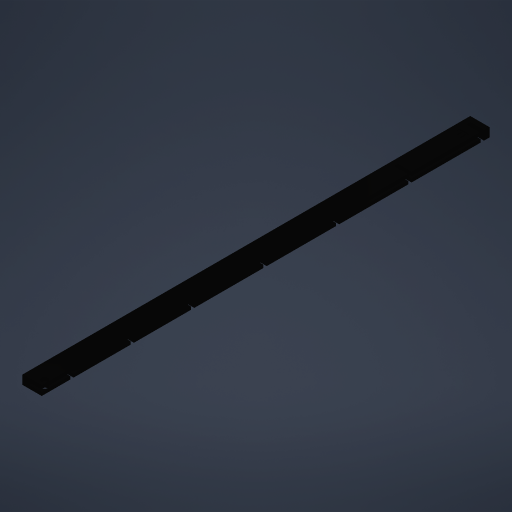
# Autodesk Inventor part: Jig_1
Saved by Autodesk Inventor 2023 (Build 270158000, 158)
## iProperties
Created: 2023-05-07
Part Number: Jig_1
Material: Generic
Document SubType Name: Modeling
Designer: szykr
Density: 1 g/cm^3
Appearance: Anodized - Black
Author: szykr
Autodesk Inventor part; units mm, degrees
ref_plane "YZ Plane" through (0, 0, 0) normal (1, 0, 0) x (0, 1, 0)
ref_plane "XZ Plane" through (0, 0, 0) normal (0, 1, 0) x (-1, 0, 0)
ref_plane "XY Plane" through (0, 0, 0) normal (0, 0, 1) x (1, 0, 0)
sketch "Sketch1" plane through (0, 0, 0) normal (0, 1, 0) x (-1, 0, 0)
  line L0 (34.2517, -400) -> (39.9859, -400) projected
  line L1 (39.9859, -398.5) -> (34.2517, -398.5) projected
  line L2 (40, -362.5) -> (40, -400) projected
  line L3 (-17.5197, -362.5) -> (39.9985, -362.5) projected
  line L4 (-17.5197, -361) -> (39.9985, -361) projected
  line L5 (-30.0427, -325) -> (39.9996, -325) projected
  line L6 (-30.0427, -323.5) -> (39.9996, -323.5) projected
  line L7 (-37.5246, -287.5) -> (39.9992, -287.5) projected
  line L8 (-37.5246, -286) -> (39.9992, -286) projected
  line L9 (-40, -250) -> (40, -250) projected
  line L10 (40, -248.5) -> (-40, -248.5) projected
  line L11 (-40, -218.75) -> (40, -218.75) projected
  line L12 (40, -217.25) -> (-40, -217.25) projected
  line L13 (-40, -187.5) -> (40, -187.5) projected
  line L14 (40, -186) -> (-40, -186) projected
  line L15 (-40, -156.25) -> (40, -156.25) projected
  line L16 (40, -154.75) -> (-40, -154.75) projected
  line L17 (-40, -125) -> (40, -125) projected
  line L18 (40, -123.5) -> (-40, -123.5) projected
  line L19 (-40, -93.75) -> (40, -93.75) projected
  line L20 (40, -92.25) -> (-40, -92.25) projected
  line L21 (-40, -62.5) -> (40, -62.5) projected
  line L22 (40, -61) -> (-40, -61) projected
  line L23 (-20.0599, -31.25) -> (40, -31.25) projected
  line L24 (40, -29.75) -> (-20.0599, -29.75) projected
  line L25 (-22.1824, 0) -> (40, 0) projected
  line L26 (40, 1.5) -> (-22.1824, 1.5) projected
  line L27 (-25.7924, 37.5) -> (37.5967, 37.5) projected
  line L28 (-25.7924, 39) -> (37.5967, 39) projected
  line L29 (-27.8365, 75) -> (30.1757, 75) projected
  line L30 (-27.8365, 76.5) -> (30.1757, 76.5) projected
  spline S0 degree 3 poles (-27.5913, 112.5) (-26.0233, 112.5) (-24.3482, 112.5) (-19.9699, 112.5) (-17.1747, 112.5) (-12.6594, 112.5) (-11.0052, 112.5) (-5.6992, 112.5) (-2.1464, 112.5) (4.6917, 112.5) (7.898, 112.5) (12.94, 112.5) (14.8552, 112.5) (17.0133, 112.5) (17.7292, 112.5) (17.4374, 112.5) (16.5312, 112.5) (13.3266, 112.5) (10.8916, 112.5) (5.1483, 112.5) (1.9055, 112.5) (-4.6814, 112.5) (-7.9404, 112.5) (-11.2251, 112.5) knots -12.727759 -12.727759 -12.727759 -12.727759 -11.944404 -11.944404 -10.775364 -10.775364 -10.102311 -10.102311 -8.634698 -8.634698 -7.023718 -7.023718 -5.528611 -5.528611 -4.394104 -4.394104 -3.316195 -3.316195 -2.113862 -2.113862 -0.985401 -0.985401 0 0 0 0 projected
  spline S1 degree 3 poles (-11.2251, 114) (-7.9404, 114) (-4.6814, 114) (1.9055, 114) (5.1483, 114) (10.8916, 114) (13.3266, 114) (16.5312, 114) (17.4374, 114) (17.7292, 114) (17.0133, 114) (14.8552, 114) (12.94, 114) (7.898, 114) (4.6917, 114) (-2.1464, 114) (-5.6992, 114) (-11.0052, 114) (-12.6594, 114) (-17.1747, 114) (-19.9699, 114) (-24.3482, 114) (-26.0233, 114) (-27.5913, 114) knots 0 0 0 0 0.985401 0.985401 2.113862 2.113862 3.316195 3.316195 4.394104 4.394104 5.528611 5.528611 7.023718 7.023718 8.634698 8.634698 10.102311 10.102311 10.775364 10.775364 11.944404 11.944404 12.727759 12.727759 12.727759 12.727759 projected
  line L31 (-40, 150) -> (0, 150) projected
  line L32 (0, 151.5) -> (-40, 151.5) projected
  line L33 (40, -325) -> (40, -361) projected
  line L34 (40, -287.5) -> (40, -323.5) projected
  line L35 (40, -250) -> (40, -286) projected
  line L36 (40, -218.75) -> (40, -248.5) projected
  line L37 (40, -187.5) -> (40, -217.25) projected
  line L38 (40, -171.125) -> (40, -186) projected
  line L39 (42.9859, -400) -> (42.9859, -171.125)
  line L40 (42.9859, -400) -> (40, -400)
  line L41 (40, -171.125) -> (42.9859, -171.125)
  line L42 (32.9859, -400) -> (32.9859, -171.125)
  line L43 (32.9859, -400) -> (40, -400)
  line L44 (32.9859, -171.125) -> (40, -171.125)
  line L45 (40, -325) -> (40, -323.5)
  line L46 (40, -287.5) -> (40, -286)
  line L47 (40, -250) -> (40, -248.5)
  line L48 (40, -218.75) -> (40, -217.25)
  line L49 (40, -187.5) -> (40, -186)
  line L50 (42.9859, -400) -> (42.9859, -403)
  line L51 (42.9859, -403) -> (32.9859, -403)
  line L52 (32.9859, -403) -> (32.9859, -400)
  line L53 (34.2517, -398.5) -> (32.9859, -398.5)
  line L54 (40, -362.5) -> (39.9985, -362.5)
  line L55 (40, -362.5) -> (40, -361)
  line L56 (39.9985, -361) -> (40, -361)
  line L57 (39.9992, -287.5) -> (40, -287.5)
  line L58 (39.9992, -286) -> (40, -286)
  line L59 (39.9996, -323.5) -> (40, -323.5)
  line L60 (39.9996, -325) -> (40, -325)
  point P0 (0, 0)
  point P1 (41.493, -400)
  dimension "d2" = 3
  dimension "d5" = 10
  dimension "d6" = 3
  constraints: 44 end point, 7 horizontal, 5 collinear, 5 perpendicular, 4 vertical, 1 horizontal alignment, 1 midpoint, 1 parallel, 1 point on line
  measures "d2" distance from line of L39 L0.end
  measures "d5" distance between parallel lines of L39 L42
  measures "d6" distance of L39.start L50.end
extrude "Extrusion1" add sketch "Sketch1" along normal mid plane 1.6 contours L0 L43 L40 L50 L51 L52 | L2 L55 L33 L45 L34 L46 L35 L47 L36 L48 L37 L49 L38 L41 L39 L40
sketch "Sketch2" plane through (0, 0.8, 0) normal (0, 1, 0) x (1, 0, 0)
  circle A0 centre (-35, 174.625) radius 1.5 projected
  line L0 (-40, 171.125) -> (-30, 171.125) projected
  line L1 (-30, 400) -> (-30, 171.125) projected
  line L2 (-40, 400) -> (-30, 400) projected
  line L3 (-40, 362.5) -> (-40, 400) projected
  line L4 (-35, 362.5) -> (-40, 362.5) projected
  line L5 (-35, 361) -> (-35, 362.5) projected
  line L6 (-40, 361) -> (-35, 361) projected
  line L7 (-40, 325) -> (-40, 361) projected
  line L8 (-34.9779, 325) -> (-40, 325) projected
  line L9 (-34.9779, 323.5) -> (-34.9779, 325) projected
  line L10 (-40, 323.5) -> (-34.9779, 323.5) projected
  line L11 (-40, 287.5) -> (-40, 323.5) projected
  line L12 (-35, 287.5) -> (-40, 287.5) projected
  line L13 (-35, 286) -> (-35, 287.5) projected
  line L14 (-40, 286) -> (-35, 286) projected
  line L15 (-40, 250) -> (-40, 286) projected
  line L16 (-35, 250) -> (-40, 250) projected
  line L17 (-35, 248.5) -> (-35, 250) projected
  line L18 (-40, 248.5) -> (-35, 248.5) projected
  line L19 (-40, 218.75) -> (-40, 248.5) projected
  line L20 (-35, 218.75) -> (-40, 218.75) projected
  line L21 (-35, 217.25) -> (-35, 218.75) projected
  line L22 (-40, 217.25) -> (-35, 217.25) projected
  line L23 (-40, 187.5) -> (-40, 217.25) projected
  line L24 (-35, 187.5) -> (-40, 187.5) projected
  line L25 (-35, 186) -> (-35, 187.5) projected
  line L26 (-40, 186) -> (-35, 186) projected
  line L27 (-40, 171.125) -> (-40, 186) projected
  line L28 (-32.9859, 403) -> (-42.9859, 403) projected
  line L29 (-42.9859, 403) -> (-42.9859, 171.125) projected
  line L30 (-32.9859, 400) -> (-32.9859, 403) projected
  line L31 (-42.9859, 171.125) -> (-40, 171.125) projected
  line L32 (-40, 400) -> (-32.9859, 400) projected
  line L33 (-32.9859, 400) -> (-32.9859, 171.125)
  line L34 (-35, 362.5) -> (-32.9859, 362.5)
  line L35 (-35, 361) -> (-32.9859, 361)
  line L36 (-34.9779, 325) -> (-32.9859, 325)
  line L37 (-34.9779, 323.5) -> (-32.9859, 323.5)
  line L38 (-35, 287.5) -> (-32.9859, 287.5)
  line L39 (-35, 286) -> (-32.9859, 286)
  line L40 (-35, 250) -> (-32.9859, 250)
  line L41 (-35, 248.5) -> (-32.9859, 248.5)
  line L42 (-35, 218.75) -> (-32.9859, 218.75)
  line L43 (-35, 217.25) -> (-32.9859, 217.25)
  line L44 (-35, 187.5) -> (-32.9859, 187.5)
  line L45 (-35, 186) -> (-32.9859, 186)
  line L46 (-40, 362.5) -> (-40, 361)
  line L47 (-40, 171.125) -> (-40, 400) projected
  line L48 (-40, 325) -> (-40, 323.5)
  line L49 (-40, 287.5) -> (-40, 286)
  line L50 (-40, 250) -> (-40, 248.5)
  line L51 (-40, 218.75) -> (-40, 217.25)
  line L52 (-40, 187.5) -> (-40, 186)
  line L53 (-39.9859, 398.5) -> (-34.2517, 398.5) projected
  line L54 (-34.2517, 398.5) -> (-32.9859, 398.5)
  line L55 (-39.9859, 398.5) -> (-40, 398.5)
  line L56 (-32.9859, 362.6) -> (-40, 362.6)
  line L57 (-40, 360.9) -> (-32.9835, 360.9)
  line L58 (-40, 325.1) -> (-32.9859, 325.1)
  line L59 (-40, 323.4) -> (-32.9859, 323.4)
  line L60 (-40, 287.6) -> (-32.9859, 287.6)
  line L61 (-40, 285.9) -> (-32.9859, 285.9)
  line L62 (-40, 250.1) -> (-32.9859, 250.1)
  line L63 (-40, 248.4) -> (-32.9859, 248.4)
  line L64 (-40, 218.85) -> (-32.9859, 218.85)
  line L65 (-40, 217.15) -> (-32.9859, 217.15)
  line L66 (-40, 187.6) -> (-32.9859, 187.6)
  line L67 (-40, 185.9) -> (-32.9859, 185.9)
  line L68 (-40, 398.4) -> (-32.9859, 398.4)
  point P0 (0, 0)
  point P1 (-32.9859, 360.9)
  dimension "d11" = 0.1
  dimension "d12" = 0.1
  dimension "d13" = 0.1
  dimension "d14" = 0.1
  dimension "d15" = 0.1
  dimension "d16" = 0.1
  dimension "d17" = 0.1
  dimension "d18" = 0.1
  dimension "d19" = 0.1
  dimension "d20" = 0.1
  dimension "d21" = 0.1
  dimension "d22" = 0.1
  dimension "d23" = 0.1
  constraints: 66 end point, 18 horizontal, 18 parallel, 3 vertical, 2 collinear, 1 perpendicular, 1 point on line, 43 other
  measures "d11" distance between parallel lines of L4 L56
  measures "d12" distance between parallel lines of L6 L57
  measures "d13" distance between parallel lines of L8 L58
  measures "d14" distance between parallel lines of L10 L59
  measures "d15" distance between parallel lines of L12 L60
  measures "d16" distance between parallel lines of L14 L61
  measures "d17" distance between parallel lines of L16 L62
  measures "d18" distance between parallel lines of L18 L63
  measures "d19" distance between parallel lines of L20 L64
  measures "d20" distance between parallel lines of L22 L65
  measures "d21" distance between parallel lines of L24 L66
  measures "d22" distance between parallel lines of L26 L67
  measures "d23" distance between parallel lines of L53 L68
extrude "Extrusion2" add sketch "Sketch2" along normal blind 1.5 contours L27 L67 L33 L0 | L31 L29 L28 L30 L2 L3 L46 L7 L47 L11 L15 L19 L23 L27 | L23 L65 L33 L66 | L33 L56 L3 L68 | L19 L63 L33 L64 | L33 L58 L7 L57 | L15 L61 L33 L62 | L33 L60 L11 L59
mirror "Mirror1" about plane through (0, 0, 0) normal (0, 1, 0) of "Extrusion2"
sketch "Sketch3" plane through (0, 2.3, 0) normal (0, 1, 0) x (1, 0, 0)
  line L0 (-40, 400) -> (-40, 401.9224)
  line L1 (-32.9859, 400) -> (-32.9859, 403) projected
  line L2 (-40, 398.4) -> (-40, 400) projected
  line L3 (-32.9859, 400) -> (-40, 400)
  line L4 (-40, 400.1) -> (-32.9859, 400.1)
  line L5 (-40, 400) -> (-32.9859, 400) projected
  point P0 (0, 0)
  dimension "d24" = 0.1
  constraints: 6 end point, 2 point on line, 1 parallel, 1 perpendicular, 1 vertical
  measures "d24" distance between parallel lines of L3 L4
extrude "Extrusion3" cut sketch "Sketch3" against normal through all
sketch "Sketch4" plane through (0, 2.3, 0) normal (0, 1, 0) x (1, 0, 0)
  line L0 (-40, 400.1) -> (-32.9859, 400.1) projected
  line L1 (-32.9859, 400.1) -> (-32.9859, 403) projected
  line L2 (-32.9859, 403) -> (-42.9859, 403) projected
  line L3 (-42.9859, 403) -> (-42.9859, 171.125) projected
  line L4 (-42.9859, 171.125) -> (-32.9859, 171.125) projected
  line L5 (-32.9859, 171.125) -> (-32.9859, 185.9) projected
  line L6 (-32.9859, 185.9) -> (-40, 185.9) projected
  line L7 (-40, 185.9) -> (-40, 187.6) projected
  line L8 (-40, 187.6) -> (-32.9859, 187.6) projected
  line L9 (-32.9859, 187.6) -> (-32.9859, 217.15) projected
  line L10 (-32.9859, 217.15) -> (-40, 217.15) projected
  line L11 (-40, 217.15) -> (-40, 218.85) projected
  line L12 (-40, 218.85) -> (-32.9859, 218.85) projected
  line L13 (-32.9859, 218.85) -> (-32.9859, 248.4) projected
  line L14 (-32.9859, 248.4) -> (-40, 248.4) projected
  line L15 (-40, 248.4) -> (-40, 250.1) projected
  line L16 (-40, 250.1) -> (-32.9859, 250.1) projected
  line L17 (-32.9859, 250.1) -> (-32.9859, 285.9) projected
  line L18 (-32.9859, 285.9) -> (-40, 285.9) projected
  line L19 (-40, 285.9) -> (-40, 287.6) projected
  line L20 (-40, 287.6) -> (-32.9859, 287.6) projected
  line L21 (-32.9859, 287.6) -> (-32.9859, 323.4) projected
  line L22 (-32.9859, 323.4) -> (-40, 323.4) projected
  line L23 (-40, 323.4) -> (-40, 325.1) projected
  line L24 (-40, 325.1) -> (-32.9859, 325.1) projected
  line L25 (-32.9859, 325.1) -> (-32.9859, 360.9) projected
  line L26 (-32.9859, 360.9) -> (-40, 360.9) projected
  line L27 (-40, 360.9) -> (-40, 362.6) projected
  line L28 (-40, 362.6) -> (-32.9859, 362.6) projected
  line L29 (-32.9859, 362.6) -> (-32.9859, 398.4) projected
  line L30 (-32.9859, 398.4) -> (-40, 398.4) projected
  line L31 (-40, 398.4) -> (-40, 400.1) projected
  circle A0 centre (-35, 174.625) radius 1.5 projected
  line L32 (-39.9859, 394.4) -> (-34.9859, 394.4)
  line L33 (-34.9859, 394.4) -> (-34.9859, 390.9)
  line L34 (-34.9859, 390.9) -> (-35.9859, 390.9)
  line L35 (-35.9859, 390.9) -> (-35.9859, 393.4)
  line L36 (-35.9859, 393.4) -> (-36.9859, 393.4)
  line L37 (-36.9859, 393.4) -> (-36.9859, 391.4)
  line L38 (-36.9859, 391.4) -> (-37.9859, 391.4)
  line L39 (-37.9859, 391.4) -> (-37.9859, 393.4)
  line L40 (-37.9859, 393.4) -> (-39.9859, 393.4)
  line L41 (-39.9859, 393.4) -> (-39.9859, 394.4)
  point P0 (0, 0)
  point P1 (-36.9859, 392.4)
  dimension "d28" = 1
  dimension "d29" = 1
  dimension "d30" = 1
  dimension "d31" = 1
  dimension "d32" = 2
  dimension "d33" = 3
  dimension "d34" = 3.5
  dimension "d35" = 4
  dimension "d36" = 3
  constraints: 20 end point, 8 perpendicular, 2 point on line, 1 horizontal, 1 midpoint
  measures "d28" distance between parallel lines of L37 L39
  measures "d29" distance between parallel lines of L35 L37
  measures "d30" distance between parallel lines of L33 L35
  measures "d31" distance between parallel lines of L40 L32
  measures "d32" distance between parallel lines of L41 L39
  measures "d33" distance between parallel lines of L32 L38
  measures "d34" distance between parallel lines of L32 L34
  measures "d35" distance between parallel lines of L30 L32
  measures "d36" distance between parallel lines of L3 L41
extrude "Extrusion4" cut sketch "Sketch4" against normal blind 0.2 contours L32 L33 L34 L35 L36 L37 L38 L39 L40 L41
equation "\"d2\" = thicc"
equation "\"d6\" = thicc"
equation "\"d11\" = slack"
equation "\"d12\" = slack"
equation "\"d13\" = slack"
equation "\"d14\" = slack"
equation "\"d15\" = slack"
equation "\"d16\" = slack"
equation "\"d17\" = slack"
equation "\"d18\" = slack"
equation "\"d19\" = slack"
equation "\"d20\" = slack"
equation "\"d21\" = slack"
equation "\"d22\" = slack"
equation "\"d23\" = slack"
equation "\"d9\" = 0.5 * thicc"
equation "\"d24\" = slack"
equation "\"thicc\" = 3"
equation "\"slack\" = 0.1"
body "Solid1"
